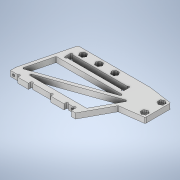
# Autodesk Inventor part: Trunk_vertical_frame_01
Saved by Autodesk Inventor 2020.4 (Build 244396000, 396)
## iProperties
Created: 2021-09-11
Part Number: Trunk_vertical_frame_01
Material: アルミニウム 2014-T4
Document SubType Name: Modeling
Designer: Masato
Density: 2.8 g/cm^3
Appearance: 滑らか - 淡い灰色
Author: Masato
Autodesk Inventor part; units mm, degrees
ref_plane "YZ Plane" through (0, 0, 0) normal (1, 0, 0) x (0, 1, 0)
ref_plane "XZ Plane" through (0, 0, 0) normal (0, 1, 0) x (-1, 0, 0)
ref_plane "XY Plane" through (0, 0, 0) normal (0, 0, 1) x (1, 0, 0)
derived "Trunk_vertical_frame_03.ipt"
sketch "スケッチ1" plane through (0, 0, 0) normal (0, 0, 1) x (1, 0, 0)
  circle A0 centre (0, 0) radius 11
  line L0 (1, 13.5) -> (28, 13.5) construction
  line L1 (28, 13.5) -> (28, -13.5) construction
  line L2 (28, -13.5) -> (1, -13.5) construction
  line L3 (1, -13.5) -> (1, 13.5) construction
  line L4 (1, 13.5) -> (28, -13.5) construction
  line L5 (28, 13.5) -> (1, -13.5) construction
  line L6 (-12, 16) -> (39.5, 16) construction
  line L7 (39.5, 16) -> (39.5, -16) construction
  line L8 (39.5, -16) -> (-12, -16) construction
  line L9 (-12, -16) -> (-12, 16) construction
  line L10 (-12, 16) -> (39.5, -16) construction
  line L11 (39.5, 16) -> (-12, -16) construction
  circle A1 centre (1, 13.5) radius 1.35
  arc A2 (0, 16) -> (-12, 10.583) centre (0, 0) ccw construction
  line L12 (-12, 0) -> (39.5, 0)
  circle A3 centre (28, 13.5) radius 1.35
  arc A4 (-12, -10.583) -> (0, -16) centre (0, 0) ccw construction
  circle A5 centre (28, -13.5) radius 1.35
  circle A6 centre (1, -13.5) radius 1.35
  arc A7 (0, 16.01) -> (-12.01, 10.5868) centre (0, 0) ccw
  line L13 (0, 16.01) -> (39.51, 16.01)
  line L14 (39.51, 16.01) -> (39.51, 13.26)
  line L15 (-12.01, 10.5868) -> (-12.01, 0)
  arc A8 (-11.4729, 11.1666) -> (-12.01, 9.8444) centre (-11.0278, 10.2156) ccw
  line L16 (-12.01, 10.5868) -> (-11.0278, 10.2156) construction
  arc A9 (39.51, 14.5251) -> (38.0251, 16.01) centre (38.7675, 15.2675) ccw
  line L17 (38.7675, 15.2675) -> (39.51, 16.01) construction
  arc A10 (38.0251, -16.01) -> (39.51, -14.5251) centre (38.7675, -15.2675) ccw
  line L18 (-12.01, -10.5868) -> (-12.01, 0)
  arc A11 (-12.01, -9.8444) -> (-11.4729, -11.1666) centre (-11.0278, -10.2156) ccw
  arc A12 (-12.01, -10.5868) -> (0, -16.01) centre (0, 0) ccw
  line L19 (0, -16.01) -> (39.51, -16.01)
  line L20 (39.51, 13.26) -> (42.01, 13.26)
  line L21 (42.01, 13.26) -> (42.01, -1.76)
  line L22 (42.01, -1.76) -> (39.51, -1.76)
  line L23 (39.51, -1.76) -> (39.51, -14.5251)
  line L24 (39.5, 13.25) -> (42, 13.25) construction
  line L25 (42, 13.25) -> (42, -1.75) construction
  line L26 (42, -1.75) -> (39.5, -1.75) construction
  line L27 (42, 5.75) -> (39.5, 5.75) construction
  arc A13 (42.01, 11.7751) -> (40.5251, 13.26) centre (41.2675, 12.5175) ccw
  line L28 (41.2675, 12.5175) -> (42.01, 13.26) construction
  arc A14 (40.5251, -1.76) -> (42.01, -0.2751) centre (41.2675, -1.0175) ccw
  circle A15 centre (-15.5, 19) radius 1.55
  line L29 (-18, 22) -> (-13, 22) construction
  line L30 (-13, 22) -> (-13, -10.5) construction
  line L31 (-13, -10.5) -> (-18, -10.5) construction
  line L32 (-18, -10.5) -> (-18, 22) construction
  line L33 (-18, 22) -> (-13, -10.5) construction
  line L34 (-13, 22) -> (-18, -10.5) construction
  line L35 (-18, 5.75) -> (-13, 5.75) construction
  line L36 (-15.5, 22) -> (-15.5, -10.5) construction
  line L37 (-18, 13.25) -> (-15.5, 13.25) construction
  line L38 (-15.5, 13.25) -> (-15.5, -1.75) construction
  line L39 (-15.5, -1.75) -> (-18, -1.75) construction
  line L40 (-18, 13.25) -> (-15.5, -1.75) construction
  line L41 (-15.5, 13.25) -> (-18, -1.75) construction
  line L42 (-15.49, -1.76) -> (-18.01, -1.76)
  line L43 (-18.01, -1.76) -> (-18.01, 13.26)
  line L44 (-18.01, 13.26) -> (-15.49, 13.26)
  line L45 (-15.49, 13.26) -> (-15.49, -1.76)
  line L46 (-15.49, -1.76) -> (-18.01, 13.26) construction
  line L47 (-18.01, -1.76) -> (-15.49, 13.26) construction
  line L48 (-16.75, 13.26) -> (-16.75, -1.76) construction
  arc A16 (-18.01, 13.26) -> (-18.01, 11.16) centre (-18.01, 12.21) ccw
  arc A17 (-15.49, 11.16) -> (-15.49, 13.26) centre (-15.49, 12.21) ccw
  arc A18 (-18.01, 0.34) -> (-18.01, -1.76) centre (-18.01, -0.71) ccw
  arc A19 (-15.49, -1.76) -> (-15.49, 0.34) centre (-15.49, -0.71) ccw
  circle A20 centre (-15.5, -7.5) radius 1.55
  line L49 (14.5, 16) -> (14.5, -16) construction
  circle A21 centre (42, 19) radius 1.55
  line L50 (39.5, 22) -> (44.5, 22) construction
  line L51 (44.5, 22) -> (44.5, -10.5) construction
  line L52 (44.5, -10.5) -> (39.5, -10.5) construction
  line L53 (39.5, 22) -> (44.5, -10.5) construction
  line L54 (44.5, 22) -> (39.5, -10.5) construction
  line L55 (42, 22) -> (42, -10.5) construction
  circle A22 centre (42, -7.5) radius 1.55
  line L56 (-12, -18.25) -> (27, -18.25) construction
  line L57 (27, -18.25) -> (27, -23.25) construction
  line L58 (27, -23.25) -> (-12, -23.25) construction
  line L59 (-12, -23.25) -> (-12, -18.25) construction
  line L60 (-12, -18.25) -> (27, -23.25) construction
  line L61 (27, -18.25) -> (-12, -23.25) construction
  line L62 (-3, -20.75) -> (18, -20.75) construction
  line L63 (18, -20.75) -> (18, -18.25) construction
  line L64 (-3, -18.25) -> (-3, -20.75) construction
  line L65 (-3, -20.75) -> (18, -18.25) construction
  line L66 (18, -20.75) -> (-3, -18.25) construction
  line L67 (-12, -20.75) -> (27, -20.75) construction
  line L68 (7.5, -18.25) -> (7.5, -23.25) construction
  line L69 (-3.01, -18.24) -> (18.01, -18.24)
  line L70 (18.01, -18.24) -> (18.01, -20.76)
  line L71 (18.01, -20.76) -> (-3.01, -20.76)
  line L72 (-3.01, -20.76) -> (-3.01, -18.24)
  line L73 (-3.01, -18.24) -> (18.01, -20.76) construction
  line L74 (18.01, -18.24) -> (-3.01, -20.76) construction
  circle A23 centre (-8, -20.75) radius 1.55
  circle A24 centre (23, -20.75) radius 1.55
  arc A25 (-0.91, -18.24) -> (-3.01, -18.24) centre (-1.96, -18.24) ccw
  arc A26 (18.01, -18.24) -> (15.91, -18.24) centre (16.96, -18.24) ccw
  line L75 (-3.01, -19.5) -> (18.01, -19.5) construction
  arc A27 (-3.01, -20.76) -> (-0.91, -20.76) centre (-1.96, -20.76) ccw
  arc A28 (15.91, -20.76) -> (18.01, -20.76) centre (16.96, -20.76) ccw
  circle A29 centre (-8, 20.75) radius 1.55
  line L76 (18.01, 20.76) -> (-3.01, 20.76)
  line L77 (-3.01, 19.5) -> (18.01, 19.5) construction
  line L78 (-3, 18.25) -> (-3, 20.75) construction
  line L79 (18, 20.75) -> (-3, 18.25) construction
  line L80 (-3, 20.75) -> (18, 18.25) construction
  line L81 (-3.01, 20.76) -> (-3.01, 18.24)
  line L82 (-3.01, 18.24) -> (18.01, 20.76) construction
  line L83 (-3.01, 18.24) -> (18.01, 18.24)
  arc A30 (-3.01, 18.24) -> (-0.91, 18.24) centre (-1.96, 18.24) ccw
  line L84 (18.01, 18.24) -> (-3.01, 20.76) construction
  line L85 (-12, 23.25) -> (-12, 18.25) construction
  arc A31 (-0.91, 20.76) -> (-3.01, 20.76) centre (-1.96, 20.76) ccw
  line L86 (7.5, 18.25) -> (7.5, 23.25) construction
  line L87 (-3, 20.75) -> (18, 20.75) construction
  line L88 (-12, 20.75) -> (27, 20.75) construction
  line L89 (27, 23.25) -> (-12, 23.25) construction
  line L90 (-12, 18.25) -> (27, 18.25) construction
  line L91 (-12, 18.25) -> (27, 23.25) construction
  line L92 (27, 18.25) -> (-12, 23.25) construction
  line L93 (27, 18.25) -> (27, 23.25) construction
  arc A32 (15.91, 18.24) -> (18.01, 18.24) centre (16.96, 18.24) ccw
  circle A33 centre (23, 20.75) radius 1.55
  line L94 (18, 20.75) -> (18, 18.25) construction
  line L95 (18.01, 18.24) -> (18.01, 20.76)
  arc A34 (18.01, 20.76) -> (15.91, 20.76) centre (16.96, 20.76) ccw
  line L96 (-18, 28.25) -> (44.5, 28.25)
  line L97 (-18, 28.25) -> (-23, 22)
  line L98 (44.5, 28.25) -> (47.5, 22)
  line L99 (-23, 22) -> (-23, -2.875)
  line L100 (47.5, 22) -> (47.5, -18.25)
  line L101 (47.5, -18.25) -> (37, -33.25)
  line L102 (-23, -2.875) -> (-33.5, -16)
  line L103 (-33.5, -16) -> (-33.5, -87)
  line L104 (37, -33.25) -> (37, -73.9)
  line L105 (37, -73.9) -> (23, -97) construction
  line L106 (23, -97) -> (-17, -97) construction
  line L107 (-17, -97) -> (-33.5, -87) construction
  circle A35 centre (-12, -92) radius 1.55
  circle A36 centre (3, -92) radius 1.55
  line L108 (-17, -97) -> (-17, -87) construction
  line L109 (-17, -87) -> (23, -87) construction
  line L110 (23, -87) -> (23, -97) construction
  line L111 (-17, -92) -> (23, -92) construction
  line L112 (3, -87) -> (3, -97) construction
  circle A37 centre (18, -92) radius 1.55
  circle A38 centre (-13.5, -58.25) radius 1.55
  line L113 (-23.5, -62.25) -> (27, -62.25)
  line L114 (27, -62.25) -> (27, -77)
  line L115 (27, -77) -> (-23.5, -77)
  line L116 (-23.5, -77) -> (-23.5, -62.25)
  line L117 (-23.5, -33.25) -> (27, -33.25)
  line L118 (27, -33.25) -> (27, -54.25)
  line L119 (27, -54.25) -> (-23.5, -54.25)
  line L120 (-23.5, -54.25) -> (-23.5, -33.25)
  circle A39 centre (-13.5, -58.25) radius 4 construction
  arc A40 (-11.4565, -94.76) -> (-9.8815, -93.8507) centre (-10.9315, -93.8507) ccw
  line L121 (-9.338, -92.9093) -> (-9.8815, -93.8507)
  arc A41 (-9.338, -92.9093) -> (-9.338, -91.0907) centre (-9.863, -92) ccw
  line L122 (-9.8815, -90.1493) -> (-9.338, -91.0907)
  arc A42 (-9.8815, -90.1493) -> (-11.4565, -89.24) centre (-10.9315, -90.1493) ccw
  line L123 (-12.5435, -89.24) -> (-11.4565, -89.24)
  arc A43 (-12.5435, -89.24) -> (-14.1185, -90.1493) centre (-13.0685, -90.1493) ccw
  line L124 (-14.662, -91.0907) -> (-14.1185, -90.1493)
  arc A44 (-14.662, -91.0907) -> (-14.662, -92.9093) centre (-14.137, -92) ccw
  line L125 (-14.1185, -93.8507) -> (-14.662, -92.9093)
  arc A45 (-14.1185, -93.8507) -> (-12.5435, -94.76) centre (-13.0685, -93.8507) ccw
  line L126 (-11.4565, -94.76) -> (-12.5435, -94.76)
  arc A46 (5.662, -92.9093) -> (5.662, -91.0907) centre (5.137, -92) ccw
  line L127 (5.1185, -90.1493) -> (5.662, -91.0907)
  line L128 (5.662, -92.9093) -> (5.1185, -93.8507)
  arc A47 (3.5435, -94.76) -> (5.1185, -93.8507) centre (4.0685, -93.8507) ccw
  arc A48 (5.1185, -90.1493) -> (3.5435, -89.24) centre (4.0685, -90.1493) ccw
  line L129 (2.4565, -89.24) -> (3.5435, -89.24)
  arc A49 (2.4565, -89.24) -> (0.8815, -90.1493) centre (1.9315, -90.1493) ccw
  line L130 (0.338, -91.0907) -> (0.8815, -90.1493)
  arc A50 (0.338, -91.0907) -> (0.338, -92.9093) centre (0.863, -92) ccw
  line L131 (0.8815, -93.8507) -> (0.338, -92.9093)
  arc A51 (0.8815, -93.8507) -> (2.4565, -94.76) centre (1.9315, -93.8507) ccw
  line L132 (3.5435, -94.76) -> (2.4565, -94.76)
  arc A52 (20.662, -92.9093) -> (20.662, -91.0907) centre (20.137, -92) ccw
  line L133 (20.1185, -90.1493) -> (20.662, -91.0907)
  line L134 (20.662, -92.9093) -> (20.1185, -93.8507)
  arc A53 (18.5435, -94.76) -> (20.1185, -93.8507) centre (19.0685, -93.8507) ccw
  arc A54 (20.1185, -90.1493) -> (18.5435, -89.24) centre (19.0685, -90.1493) ccw
  line L135 (17.4565, -89.24) -> (18.5435, -89.24)
  arc A55 (17.4565, -89.24) -> (15.8815, -90.1493) centre (16.9315, -90.1493) ccw
  line L136 (15.338, -91.0907) -> (15.8815, -90.1493)
  arc A56 (15.338, -91.0907) -> (15.338, -92.9093) centre (15.863, -92) ccw
  line L137 (15.8815, -93.8507) -> (15.338, -92.9093)
  arc A57 (15.8815, -93.8507) -> (17.4565, -94.76) centre (16.9315, -93.8507) ccw
  line L138 (18.5435, -94.76) -> (17.4565, -94.76)
  line L139 (-33.5, -87) -> (46, -87)
  line L140 (46, -87) -> (46, -117) construction
  line L141 (46, -117) -> (33, -141)
  line L142 (-33.5, -87) -> (-33.5, -139)
  line L143 (-33.5, -139) -> (28.01, -139)
  arc A58 (-24.5, -139) -> (-26.6, -139) centre (-25.55, -139) ccw
  line L144 (-24.5, -139) -> (-24.5, -141)
  line L145 (-14.5, -141) -> (-14.5, -139)
  arc A59 (-12.4, -139) -> (-14.5, -139) centre (-13.45, -139) ccw
  arc A60 (6.5, -139) -> (4.4, -139) centre (5.45, -139) ccw
  line L146 (6.5, -139) -> (6.5, -141)
  line L147 (19, -141) -> (19, -139)
  arc A61 (21.1, -139) -> (19, -139) centre (20.05, -139) ccw
  line L148 (-30.5, -139) -> (-30.5, -141) construction
  line L149 (-33.5, -139) -> (-33.5, -141) construction
  line L150 (-24.5, -141) -> (-14.5, -141)
  line L151 (28, -139) -> (28, -141) construction
  line L152 (6.5, -141) -> (19, -141)
  line L153 (25, -139) -> (25, -141) construction
  line L154 (-33.5, -141) -> (19, -141) construction
  line L155 (19, -141) -> (33, -141) construction
  line L156 (28.01, -139) -> (34.0833, -139) construction
  arc A62 (28.01, -139) -> (25.91, -139) centre (26.96, -139) ccw
  line L157 (-19, -97) -> (36.5, -97) construction
  line L158 (36.5, -97) -> (36.5, -102) construction
  line L159 (36.5, -102) -> (-19, -102) construction
  line L160 (-19, -102) -> (-19, -97) construction
  line L161 (-19, -99.5) -> (36.5, -99.5) construction
  line L162 (8.75, -97) -> (8.75, -102) construction
  line L163 (-19.05, -96.95) -> (36.55, -96.95)
  line L164 (36.55, -96.95) -> (36.55, -102.05)
  line L165 (36.55, -102.05) -> (-19.05, -102.05)
  line L166 (-19.05, -102.05) -> (-19.05, -96.95)
  line L167 (-19.05, -96.95) -> (36.55, -102.05) construction
  line L168 (36.55, -96.95) -> (-19.05, -102.05) construction
  arc A63 (-16.95, -96.95) -> (-19.05, -96.95) centre (-18, -96.95) ccw
  arc A64 (36.55, -96.95) -> (34.45, -96.95) centre (35.5, -96.95) ccw
  arc A65 (-19.05, -102.05) -> (-16.95, -102.05) centre (-18, -102.05) ccw
  arc A66 (34.45, -102.05) -> (36.55, -102.05) centre (35.5, -102.05) ccw
  line L169 (46, -87) -> (68.5, -90.0728)
  line L170 (68.5, -90.0728) -> (68.5, -113.9272)
  line L171 (68.5, -113.9272) -> (46, -117)
  line L172 (46, -102) -> (68.5, -102) construction
  circle A67 centre (64, -94) radius 4.5 construction
  line L173 (64, -94) -> (64, -102) construction
  circle A68 centre (64, -94) radius 2.25
  line L174 (64, -97.187) -> (61.24, -95.5935)
  line L175 (61.24, -95.5935) -> (61.24, -92.4065)
  line L176 (61.24, -92.4065) -> (64, -90.813)
  line L177 (64, -90.813) -> (66.76, -92.4065)
  line L178 (66.76, -92.4065) -> (66.76, -95.5935)
  line L179 (66.76, -95.5935) -> (64, -97.187)
  arc A69 (63.0907, -96.662) -> (64.9093, -96.662) centre (64, -96.137) ccw
  arc A70 (65.8507, -96.1185) -> (66.76, -94.5435) centre (65.8507, -95.0685) ccw
  arc A71 (66.76, -93.4565) -> (65.8507, -91.8815) centre (65.8507, -92.9315) ccw
  arc A72 (64.9093, -91.338) -> (63.0907, -91.338) centre (64, -91.863) ccw
  arc A73 (62.1493, -91.8815) -> (61.24, -93.4565) centre (62.1493, -92.9315) ccw
  arc A74 (61.24, -94.5435) -> (62.1493, -96.1185) centre (62.1493, -95.0685) ccw
  circle A75 centre (64, -110) radius 2.25
  line L180 (64, -106.813) -> (61.24, -108.4065)
  line L181 (61.24, -108.4065) -> (61.24, -111.5935)
  line L182 (61.24, -111.5935) -> (64, -113.187)
  line L183 (64, -113.187) -> (66.76, -111.5935)
  line L184 (66.76, -111.5935) -> (66.76, -108.4065)
  line L185 (66.76, -108.4065) -> (64, -106.813)
  arc A76 (64.9093, -107.338) -> (63.0907, -107.338) centre (64, -107.863) ccw
  arc A77 (66.76, -109.4565) -> (65.8507, -107.8815) centre (65.8507, -108.9315) ccw
  arc A78 (65.8507, -112.1185) -> (66.76, -110.5435) centre (65.8507, -111.0685) ccw
  arc A79 (63.0907, -112.662) -> (64.9093, -112.662) centre (64, -112.137) ccw
  arc A80 (61.24, -110.5435) -> (62.1493, -112.1185) centre (62.1493, -111.0685) ccw
  arc A81 (62.1493, -107.8815) -> (61.24, -109.4565) centre (62.1493, -108.9315) ccw
  line L186 (47.4794, -107.97) -> (33.3798, -134)
  line L187 (33.3798, -134) -> (-25.9193, -134)
  line L188 (-25.9193, -134) -> (47.4794, -107.97)
  line L189 (-29.9688, -132.253) -> (44.0587, -106)
  line L190 (44.0587, -106) -> (-23.3824, -106)
  line L191 (-23.3824, -106) -> (-29.9688, -132.253)
  line L192 (-21.7087, -87) -> (-33.5, -134)
  line L193 (-30.407, -134) -> (48.5465, -106) construction
  line L194 (-25.9193, -134) -> (-33.5, -134) construction
  line L195 (28.01, -143) -> (31.9167, -143)
  line L196 (28.01, -139) -> (28.01, -143)
  line L197 (33, -141) -> (31.9167, -143)
  point P0 (14.5, 0)
  point P1 (-15.5, 5.75)
  point P2 (-16.75, 5.75)
  point P3 (14.5, 0)
  point P4 (42, 5.75)
  point P5 (42, 5.75)
  point P6 (7.5, -20.75)
  point P7 (7.5, -19.5)
  point P8 (7.5, -19.5)
  point P9 (7.5, -19.5)
  point P10 (7.5, -19.5)
  point P11 (7.5, 20.75)
  point P12 (7.5, 19.5)
  point P13 (7.5, 19.5)
  point P14 (7.5, 19.5)
  point P15 (7.5, 19.5)
  point P16 (3, -89.25)
  point P17 (-10.4065, -94.76)
  point P18 (-8.813, -92)
  point P19 (-10.4065, -89.24)
  point P20 (-13.5935, -89.24)
  point P21 (-13.5935, -89.24)
  point P22 (-15.187, -92)
  point P23 (-13.5935, -94.76)
  point P24 (-15.187, -92)
  point P25 (-8.813, -92)
  point P26 (3, -92)
  point P27 (6.187, -92)
  point P28 (6.187, -92)
  point P29 (4.5935, -89.24)
  point P30 (4.5935, -94.76)
  point P31 (3, -92)
  point P32 (3, -92)
  point P33 (1.4065, -89.24)
  point P34 (1.4065, -89.24)
  point P35 (-0.187, -92)
  point P36 (-0.187, -92)
  point P37 (1.4065, -94.76)
  point P38 (18, -92)
  point P39 (21.187, -92)
  point P40 (21.187, -92)
  point P41 (19.5935, -89.24)
  point P42 (19.5935, -94.76)
  point P43 (18, -92)
  point P44 (18, -92)
  point P45 (16.4065, -89.24)
  point P46 (16.4065, -89.24)
  point P47 (14.813, -92)
  point P48 (14.813, -92)
  point P49 (16.4065, -94.76)
  point P50 (3, -87)
  point P51 (8.75, -99.5)
  point P52 (66.76, -95.5935)
  point P53 (66.76, -92.4065)
  point P54 (64, -90.813)
  point P55 (61.24, -92.4065)
  point P56 (66.76, -111.5935)
  point P57 (64, -113.187)
  point P58 (61.24, -111.5935)
  point P59 (34.45, -102.05)
  point P60 (-16.95, -102.05)
  point P61 (34.45, -96.95)
  point P62 (-14.1185, -90.1493)
  point P63 (0.8815, -90.1493)
  point P64 (15.8815, -90.1493)
  point P65 (65.8507, -112.1185)
  point P66 (64.9093, -112.662)
  point P67 (63.0907, -112.662)
  point P68 (62.1493, -112.1185)
  point P69 (61.24, -110.5435)
  point P70 (61.24, -109.4565)
  point P71 (62.1493, -107.8815)
  point P72 (65.8507, -107.8815)
  point P73 (66.76, -109.4565)
  point P74 (66.76, -110.5435)
  point P75 (61.24, -94.5435)
  point P76 (61.24, -93.4565)
  point P77 (62.1493, -91.8815)
  point P78 (63.0907, -91.338)
  point P79 (64.9093, -91.338)
  point P80 (65.8507, -91.8815)
  point P81 (66.76, -93.4565)
  point P82 (66.76, -94.5435)
  point P83 (65.8507, -96.1185)
  point P84 (62.1493, -96.1185)
  dimension "d1" = 30
  dimension "d2" = 1.05
  dimension "d3" = 1.05
  dimension "d4" = 10
  dimension "d5" = 12.5
  dimension "d6" = 1.05
  dimension "d7" = 1.05
  dimension "d9" = 6
  dimension "d12" = 2
  dimension "d16" = 3
  dimension "d17" = 3
  dimension "d18" = 6
  dimension "d20" = 21
  dimension "d21" = 61.5
  dimension "d22" = 5
  dimension "d23" = 1.05
  dimension "d24" = 42
  dimension "d25" = 43
  dimension "d27" = 0.05
  dimension "d28" = 0.05
  dimension "d29" = 5
  dimension "d30" = 55.5
  dimension "d31" = 1.05
  dimension "d33" = 22
  dimension "d34" = 9
  dimension "d35" = 18
  dimension "d36" = 4.5
  dimension "d37" = 5.52
  dimension "d38" = 1.05
  dimension "d41" = 360
  dimension "d43" = 16
  dimension "d44" = 3
  dimension "d47" = 5
  dimension "d48" = 4
  dimension "d50" = 3
  dimension "d52" = 1.5
  dimension "d53" = 1.5
  dimension "d55" = 5
  dimension "d73" = 5
  dimension "d74" = 4
  dimension "d75" = 0.01
  measures "d1" distance of L140.end L139.end
  measures "d2" radius of A58
  measures "d3" radius of A60
  measures "d4" distance of L145.start L144.end
  measures "d5" distance of L147.start L146.end
  measures "d6" radius of A59
  measures "d7" radius of A61
  measures "d9" distance of L144.end L148.end
  measures "d12" distance of L142.end L149.end
  measures "d16" distance of L149.end L148.end
  measures "d17" distance of L151.end L153.end
  measures "d18" distance of L147.start L153.end
  measures "d20" distance of L146.end L145.start
  measures "d21" distance of L149.end L151.end
  measures "d22" distance of L141.end L151.end
  measures "d23" radius of A62
  measures "d24" vertical distance of L142.end L106.end
  measures "d25" distance of L139.end L112.start
  measures "d27" horizontal distance of L163.start L157.start
  measures "d28" horizontal distance of L157.start L163.start
  measures "d29" distance of L159.end L157.start
  measures "d30" distance of L161.end L161.start
  measures "d31" radius of A63
  measures "d33" horizontal distance of L157.start point (3, -92)
  measures "d34" diameter of A67
  measures "d35" distance of L172.start L173.end
  measures "d36" diameter of A68
  measures "d37" distance from line of L176 L178.end
  measures "d38" radius of A69
  measures "d43" distance of point (64, -110) A68.centre
  measures "d44" distance between parallel lines of L141 L186
  measures "d47" distance of L192.end L142.end
  measures "d48" vertical distance of L190.end L159.end
  measures "d50" distance between parallel lines of L192 L191
  measures "d52" distance between parallel lines of L188 L193
  measures "d53" distance between parallel lines of L193 L189
  measures "d55" distance from line of L163.start L192
  measures "d73" vertical distance of A35.centre L157.start
  measures "d74" distance between parallel lines of L195 L156
  measures "d75" distance between parallel lines of L196 L151
extrude "押し出し1" add sketch "スケッチ1" along normal blind 5 contours L139 L169 L170 L171 L141 L197 L195 L196 A62 L143 A61 A60 A59 A58 L142 L192 | L143 L145 L150 L144 | L143 L147 L152 L146
sketch "スケッチ2" plane through (-33.5, -139, 0) normal (0, -1, 0) x (1, 0, 0)
  line L0 (52.5, 0) -> (52.5, 5) projected
  point P0 (33.5, 0)
  point P1 (3, 2.5)
  point P2 (0, 0)
  point P3 (58.5, 2.5)
  dimension "d58" = 3
  dimension "d59" = 2.5
  dimension "d60" = 6
  dimension "d61" = 2.5
  measures "d58" horizontal distance of point (0, 0) point (3, 2.5)
  measures "d59" vertical distance of point (0, 0) point (3, 2.5)
  measures "d60" distance from line of L0 point (58.5, 2.5)
  measures "d61" vertical distance of point (0, 0) point (58.5, 2.5)
hole "穴1" at (-30.5, -139, 2.5) at (25, -139, 2.5) direction (0, 1, 0) diameter 2.459 depth 5 thread size "M3x0.5" class "6H" standard "ISO Metric profile"
fillet "フィレット1" radius 1 6 edges at (-21.7087, -87, 2.5) (68.5, -90.0728, 2.5) (68.5, -113.9272, 2.5) (46, -117, 2.5) (46, -87, 2.5) (-33.5, -134, 2.5)
extrude "押し出し2" add sketch "スケッチ1" along normal blind 2.8 contours A69 L174 | L174 L175 L176 L177 L178 L179 | L179 A69 | A74 L174 | L179 A70 | A74 L175 | L178 A70 | A73 L175 | L178 A71 | A73 L176 | L177 A71 | A72 L176 | L177 A72 | L185 L184 L183 L182 L181 L180 | A76 L185 | L180 A76 | L180 A81 | A77 L185 | L181 A81 | A77 L184 | L181 A80 | A78 L184 | L182 A80 | A78 L183 | L182 A79 | A79 L183
fillet "フィレット2" radius 1 6 edges at (-23.3824, -106, 2.5) (-29.9688, -132.253, 2.5) (-25.9193, -134, 2.5) (44.0587, -106, 2.5) (33.3798, -134, 2.5) (47.4794, -107.97, 2.5)
equation "\"d3\" = d2"
equation "\"d6\" = d2"
equation "\"d7\" = d2"
equation "\"d23\" = d7"
equation "\"d28\" = d27"
equation "\"d31\" = d2"
equation "\"d38\" = d2"
equation "\"d50\" = d49"
equation "\"d13\" = d10"
equation "\"d49\" = 3"
equation "\"d10\" = 0.01"
